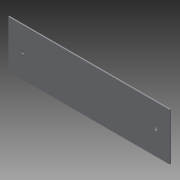
# Autodesk Inventor part: tabliczka z autorami i opiekunem na przod 170 x 50
Saved by Autodesk Inventor 2014 (Build 180170000, 170)
## iProperties
Created: 2018-03-25
Part Number: tabliczka z autorami i opiekunem na przod 170 x 50
Material: Generic
Document SubType Name: Modeling
Designer: HP820
Density: 1 g/cm^3
Appearance: Default
Author: HP820
Autodesk Inventor part; units mm, degrees
(part 1 of 3)
ref_plane "YZ Plane" through (0, 0, 0) normal (1, 0, 0) x (0, 1, 0)
ref_plane "XZ Plane" through (0, 0, 0) normal (0, 1, 0) x (-1, 0, 0)
ref_plane "XY Plane" through (0, 0, 0) normal (0, 0, 1) x (1, 0, 0)
sketch "Sketch1" plane through (0, 0, 0) normal (0, 1, 0) x (-1, 0, 0)
  line L0 (-85, 25) -> (85, 25)
  line L1 (85, 25) -> (85, -25)
  line L2 (85, -25) -> (-85, -25)
  line L3 (-85, -25) -> (-85, 25)
  line L4 (-85, 25) -> (85, -25) construction
  line L5 (85, 25) -> (-85, -25) construction
  point P0 (0, 0)
  dimension "d0" = 170
  dimension "d1" = 50
  constraints: 12 end point, 2 midpoint, 2 parallel, 1 horizontal, 1 perpendicular
  measures "d0" distance of L1.end L2.end
  measures "d1" distance of L0.end L1.end
extrude "Extrusion1" add sketch "Sketch1" along normal blind 1.2
sketch "Sketch2" plane through (0, 1.2, 0) normal (0, 1, 0) x (1, 0, 0)
  line L0 (-82.9131, 23.4055) -> (83.5665, 23.4055) construction
  line L1 (83.5665, 23.4055) -> (83.5665, -23.9623) construction
  line L2 (83.5665, -23.9623) -> (-82.9131, -23.9623) construction
  line L3 (-82.9131, -23.9623) -> (-82.9131, 23.4055) construction
  spline S0 degree 2 poles (-28.4034, 19.5042) (-28.4034, 19.1209) (-28.6486, 18.4256) (-28.8759, 18.1938) knots 0 0 0 1 2 2 2
  spline S1 degree 2 poles (-28.8759, 18.1938) (-29.0141, 18.0467) (-29.3528, 17.8061) (-29.5534, 17.7214) knots 0 0 0 1 2 2 2
  spline S2 degree 2 poles (-29.5534, 17.7214) (-29.7584, 17.6367) (-30.2353, 17.5386) (-30.5295, 17.5386) knots 0 0 0 1 2 2 2
  line L4 (-30.5295, 17.5386) -> (-31.2515, 17.5386)
  line L5 (-31.2515, 17.5386) -> (-31.2515, 15.738)
  line L6 (-31.2515, 15.738) -> (-32.6332, 15.738)
  line L7 (-32.6332, 15.738) -> (-32.6332, 21.238)
  line L8 (-32.6332, 21.238) -> (-30.4983, 21.238)
  spline S3 degree 2 poles (-30.4983, 21.238) (-30.0258, 21.238) (-29.335, 21.0642) (-29.0542, 20.877) knots 0 0 0 1 2 2 2
  spline S4 degree 2 poles (-29.0542, 20.877) (-28.7422, 20.6675) (-28.4034, 19.9811) (-28.4034, 19.5042) knots 0 0 0 1 2 2 2
  spline S5 degree 2 poles (-29.8208, 19.4685) (-29.8208, 19.7048) (-30.0436, 20.039) (-30.1952, 20.1014) knots 0 0 0 1 2 2 2
  spline S6 degree 2 poles (-30.1952, 20.1014) (-30.3913, 20.1861) (-30.7479, 20.2129) (-31.0554, 20.2129) knots 0 0 0 1 2 2 2
  line L9 (-31.0554, 20.2129) -> (-31.2515, 20.2129)
  line L10 (-31.2515, 20.2129) -> (-31.2515, 18.5638)
  line L11 (-31.2515, 18.5638) -> (-31.1534, 18.5638)
  spline S7 degree 2 poles (-31.1534, 18.5638) (-30.9618, 18.5638) (-30.6141, 18.5727) (-30.4849, 18.595) knots 0 0 0 1 2 2 2
  spline S8 degree 2 poles (-30.4849, 18.595) (-30.3735, 18.6128) (-30.1283, 18.7197) (-30.0615, 18.7866) knots 0 0 0 1 2 2 2
  spline S9 degree 2 poles (-30.0615, 18.7866) (-29.9188, 18.9203) (-29.8208, 19.2189) (-29.8208, 19.4685) knots 0 0 0 1 2 2 2
  line L12 (-24.9537, 18.6618) -> (-25.0607, 18.6618)
  spline S10 degree 2 poles (-25.0607, 18.6618) (-25.1364, 18.6886) (-25.4172, 18.7153) (-25.5866, 18.7153) knots 0 0 0 1 2 2 2
  spline S11 degree 2 poles (-25.5866, 18.7153) (-25.7872, 18.7153) (-26.2373, 18.595) (-26.4468, 18.5147) knots 0 0 0 1 2 2 2
  line L13 (-26.4468, 18.5147) -> (-26.4468, 15.738)
  line L14 (-26.4468, 15.738) -> (-27.7393, 15.738)
  line L15 (-27.7393, 15.738) -> (-27.7393, 19.8875)
  line L16 (-27.7393, 19.8875) -> (-26.4468, 19.8875)
  line L17 (-26.4468, 19.8875) -> (-26.4468, 19.2903)
  spline S12 degree 2 poles (-26.4468, 19.2903) (-26.3577, 19.3705) (-26.0457, 19.6201) (-25.9164, 19.6958) knots 0 0 0 1 2 2 2
  spline S13 degree 2 poles (-25.9164, 19.6958) (-25.7738, 19.7805) (-25.3994, 19.9009) (-25.2345, 19.9009) knots 0 0 0 1 2 2 2
  spline S14 degree 2 poles (-25.2345, 19.9009) (-25.1721, 19.9009) (-25.0161, 19.892) (-24.9537, 19.8875) knots 0 0 0 1 2 2 2
  line L18 (-24.9537, 19.8875) -> (-24.9537, 18.6618)
  spline S15 degree 2 poles (-20.4788, 17.8105) (-20.4788, 16.7854) (-21.5975, 15.6087) (-22.6182, 15.6087) knots 0 0 0 1 2 2 2
  spline S16 degree 2 poles (-22.6182, 15.6087) (-23.6344, 15.6087) (-24.762, 16.7854) (-24.762, 17.8105) knots 0 0 0 1 2 2 2
  spline S17 degree 2 poles (-24.762, 17.8105) (-24.762, 18.8445) (-23.6344, 20.0168) (-22.6182, 20.0168) knots 0 0 0 1 2 2 2
  spline S18 degree 2 poles (-22.6182, 20.0168) (-21.602, 20.0168) (-20.4788, 18.8401) (-20.4788, 17.8105) knots 0 0 0 1 2 2 2
  spline S19 degree 2 poles (-21.8026, 17.8016) (-21.8026, 18.1715) (-21.9229, 18.6663) (-22.0299, 18.8133) knots 0 0 0 1 2 2 2
  spline S20 degree 2 poles (-22.0299, 18.8133) (-22.1457, 18.9693) (-22.4355, 19.0897) (-22.6182, 19.0897) knots 0 0 0 1 2 2 2
  spline S21 degree 2 poles (-22.6182, 19.0897) (-22.7965, 19.0897) (-23.0773, 18.9827) (-23.1932, 18.8312) knots 0 0 0 1 2 2 2
  spline S22 degree 2 poles (-23.1932, 18.8312) (-23.3046, 18.6886) (-23.4383, 18.1849) (-23.4383, 17.8016) knots 0 0 0 1 2 2 2
  spline S23 degree 2 poles (-23.4383, 17.8016) (-23.4383, 17.4227) (-23.3135, 16.9548) (-23.211, 16.8121) knots 0 0 0 1 2 2 2
  spline S24 degree 2 poles (-23.211, 16.8121) (-23.1085, 16.6695) (-22.7965, 16.5358) (-22.6093, 16.5358) knots 0 0 0 1 2 2 2
  spline S25 degree 2 poles (-22.6093, 16.5358) (-22.4533, 16.5358) (-22.1324, 16.6695) (-22.0343, 16.8032) knots 0 0 0 1 2 2 2
  spline S26 degree 2 poles (-22.0343, 16.8032) (-21.9229, 16.9592) (-21.8026, 17.4094) (-21.8026, 17.8016) knots 0 0 0 1 2 2 2
  spline S27 degree 2 poles (-18.0363, 15.6667) (-18.0363, 14.9625) (-18.8698, 14.178) (-19.5295, 14.178) knots 0 0 0 1 2 2 2
  spline S28 degree 2 poles (-19.5295, 14.178) (-19.886, 14.178) (-20.461, 14.2404) (-20.5947, 14.2761) knots 0 0 0 1 2 2 2
  line L19 (-20.5947, 14.2761) -> (-20.5947, 15.2299)
  line L20 (-20.5947, 15.2299) -> (-20.4966, 15.2299)
  spline S29 degree 2 poles (-20.4966, 15.2299) (-20.3674, 15.1898) (-20.0643, 15.1407) (-19.9707, 15.1407) knots 0 0 0 1 2 2 2
  spline S30 degree 2 poles (-19.9707, 15.1407) (-19.5963, 15.1407) (-19.3289, 15.5998) (-19.3289, 16.1213) knots 0 0 0 1 2 2 2
  line L21 (-19.3289, 16.1213) -> (-19.3289, 18.9872)
  line L22 (-19.3289, 18.9872) -> (-20.0732, 18.9872)
  line L23 (-20.0732, 18.9872) -> (-20.0732, 19.8875)
  line L24 (-20.0732, 19.8875) -> (-18.0363, 19.8875)
  line L25 (-18.0363, 19.8875) -> (-18.0363, 15.6667)
  line L26 (-18.0363, 20.4803) -> (-19.4136, 20.4803)
  line L27 (-19.4136, 20.4803) -> (-19.4136, 21.4876)
  line L28 (-19.4136, 21.4876) -> (-18.0363, 21.4876)
  line L29 (-18.0363, 21.4876) -> (-18.0363, 20.4803)
  spline S31 degree 2 poles (-14.9209, 15.6266) (-16.0975, 15.6266) (-17.35, 16.7497) (-17.35, 17.7882) knots 0 0 0 1 2 2 2
  spline S32 degree 2 poles (-17.35, 17.7882) (-17.35, 18.8044) (-16.1822, 20.0168) (-15.1303, 20.0168) knots 0 0 0 1 2 2 2
  spline S33 degree 2 poles (-15.1303, 20.0168) (-14.181, 20.0168) (-13.2183, 18.9872) (-13.2183, 18.0334) knots 0 0 0 1 2 2 2
  line L30 (-13.2183, 18.0334) -> (-13.2183, 17.5654)
  line L31 (-13.2183, 17.5654) -> (-16.0574, 17.5654)
  spline S34 degree 2 poles (-16.0574, 17.5654) (-16.0396, 17.2757) (-15.8301, 16.8924) (-15.6607, 16.7765) knots 0 0 0 1 2 2 2
  spline S35 degree 2 poles (-15.6607, 16.7765) (-15.4958, 16.6606) (-15.0501, 16.5625) (-14.7872, 16.5625) knots 0 0 0 1 2 2 2
  spline S36 degree 2 poles (-14.7872, 16.5625) (-14.5643, 16.5625) (-14.1275, 16.6606) (-13.9448, 16.7453) knots 0 0 0 1 2 2 2
  spline S37 degree 2 poles (-13.9448, 16.7453) (-13.7843, 16.8121) (-13.5169, 16.977) (-13.4322, 17.0394) knots 0 0 0 1 2 2 2
  line L32 (-13.4322, 17.0394) -> (-13.294, 17.0394)
  line L33 (-13.294, 17.0394) -> (-13.294, 15.9697)
  spline S38 degree 2 poles (-13.294, 15.9697) (-13.4545, 15.9074) (-13.713, 15.8004) (-13.9448, 15.7469) knots 0 0 0 1 2 2 2
  spline S39 degree 2 poles (-13.9448, 15.7469) (-14.1543, 15.689) (-14.6, 15.6266) (-14.9209, 15.6266) knots 0 0 0 1 2 2 2
  spline S40 degree 2 poles (-14.493, 18.3454) (-14.5019, 18.7554) (-14.8629, 19.1877) (-15.2329, 19.1877) knots 0 0 0 1 2 2 2
  spline S41 degree 2 poles (-15.2329, 19.1877) (-15.6117, 19.1877) (-16.0396, 18.7331) (-16.0619, 18.3454) knots 0 0 0 1 2 2 2
  line L34 (-16.0619, 18.3454) -> (-14.493, 18.3454)
  line L35 (-8.4002, 15.738) -> (-9.9379, 15.738)
  line L36 (-9.9379, 15.738) -> (-11.0611, 17.5386)
  line L37 (-11.0611, 17.5386) -> (-11.2616, 17.2712)
  line L38 (-11.2616, 17.2712) -> (-11.2616, 15.738)
  line L39 (-11.2616, 15.738) -> (-12.5542, 15.738)
  line L40 (-12.5542, 15.738) -> (-12.5542, 21.4831)
  line L41 (-12.5542, 21.4831) -> (-11.2616, 21.4831)
  line L42 (-11.2616, 21.4831) -> (-11.2616, 18.2651)
  line L43 (-11.2616, 18.2651) -> (-10.0359, 19.8875)
  line L44 (-10.0359, 19.8875) -> (-8.5072, 19.8875)
  line L45 (-8.5072, 19.8875) -> (-9.9602, 18.1002)
  line L46 (-9.9602, 18.1002) -> (-8.4002, 15.738)
  spline S42 degree 2 poles (-6.4079, 15.6578) (-7.1968, 15.6578) (-7.9188, 16.3085) (-7.9188, 17.0484) knots 0 0 0 1 2 2 2
  line L47 (-7.9188, 17.0484) -> (-7.9188, 18.9872)
  line L48 (-7.9188, 18.9872) -> (-8.4136, 18.9872)
  line L49 (-8.4136, 18.9872) -> (-8.4136, 19.8875)
  line L50 (-8.4136, 19.8875) -> (-7.9188, 19.8875)
  line L51 (-7.9188, 19.8875) -> (-7.9188, 21.0731)
  line L52 (-7.9188, 21.0731) -> (-6.6263, 21.0731)
  line L53 (-6.6263, 21.0731) -> (-6.6263, 19.8875)
  line L54 (-6.6263, 19.8875) -> (-5.3783, 19.8875)
  line L55 (-5.3783, 19.8875) -> (-5.3783, 18.9872)
  line L56 (-5.3783, 18.9872) -> (-6.6263, 18.9872)
  line L57 (-6.6263, 18.9872) -> (-6.6263, 17.5119)
  spline S43 degree 2 poles (-6.6263, 17.5119) (-6.6263, 17.2935) (-6.6174, 16.9681) (-6.5639, 16.8389) knots 0 0 0 1 2 2 2
  spline S44 degree 2 poles (-6.5639, 16.8389) (-6.5104, 16.7096) (-6.2474, 16.5581) (-5.9979, 16.5581) knots 0 0 0 1 2 2 2
  spline S45 degree 2 poles (-5.9979, 16.5581) (-5.8909, 16.5581) (-5.5566, 16.6472) (-5.4897, 16.6829) knots 0 0 0 1 2 2 2
  line L58 (-5.4897, 16.6829) -> (-5.3783, 16.6829)
  line L59 (-5.3783, 16.6829) -> (-5.3783, 15.7736)
  spline S46 degree 2 poles (-5.3783, 15.7736) (-5.5878, 15.7202) (-6.0602, 15.6578) (-6.4079, 15.6578) knots 0 0 0 1 2 2 2
  line L60 (3.5447, 19.8875) -> (2.3324, 15.738)
  line L61 (2.3324, 15.738) -> (0.9596, 15.738)
  line L62 (0.9596, 15.738) -> (0.2286, 18.4211)
  line L63 (0.2286, 18.4211) -> (-0.5023, 15.738)
  line L64 (-0.5023, 15.738) -> (-1.8751, 15.738)
  line L65 (-1.8751, 15.738) -> (-3.0785, 19.8875)
  line L66 (-3.0785, 19.8875) -> (-1.7191, 19.8875)
  line L67 (-1.7191, 19.8875) -> (-1.0817, 17.142)
  line L68 (-1.0817, 17.142) -> (-0.2973, 19.8875)
  line L69 (-0.2973, 19.8875) -> (0.8482, 19.8875)
  line L70 (0.8482, 19.8875) -> (1.588, 17.142)
  line L71 (1.588, 17.142) -> (2.2165, 19.8875)
  line L72 (2.2165, 19.8875) -> (3.5447, 19.8875)
  line L73 (7.9616, 19.8875) -> (5.8713, 14.2181)
  line L74 (5.8713, 14.2181) -> (4.4807, 14.2181)
  line L75 (4.4807, 14.2181) -> (5.1091, 15.8405)
  line L76 (5.1091, 15.8405) -> (3.5893, 19.8875)
  line L77 (3.5893, 19.8875) -> (4.9442, 19.8875)
  line L78 (4.9442, 19.8875) -> (5.8178, 17.2846)
  line L79 (5.8178, 17.2846) -> (6.6334, 19.8875)
  line L80 (6.6334, 19.8875) -> (7.9616, 19.8875)
  line L81 (12.6014, 15.738) -> (11.0637, 15.738)
  line L82 (11.0637, 15.738) -> (9.9406, 17.5386)
  line L83 (9.9406, 17.5386) -> (9.74, 17.2712)
  line L84 (9.74, 17.2712) -> (9.74, 15.738)
  line L85 (9.74, 15.738) -> (8.4474, 15.738)
  line L86 (8.4474, 15.738) -> (8.4474, 21.4831)
  line L87 (8.4474, 21.4831) -> (9.74, 21.4831)
  line L88 (9.74, 21.4831) -> (9.74, 18.2651)
  line L89 (9.74, 18.2651) -> (10.9657, 19.8875)
  line L90 (10.9657, 19.8875) -> (12.4945, 19.8875)
  line L91 (12.4945, 19.8875) -> (11.0415, 18.1002)
  line L92 (11.0415, 18.1002) -> (12.6014, 15.738)
  spline S47 degree 2 poles (16.9872, 17.8105) (16.9872, 16.7854) (15.8684, 15.6087) (14.8478, 15.6087) knots 0 0 0 1 2 2 2
  spline S48 degree 2 poles (14.8478, 15.6087) (13.8316, 15.6087) (12.7039, 16.7854) (12.7039, 17.8105) knots 0 0 0 1 2 2 2
  spline S49 degree 2 poles (12.7039, 17.8105) (12.7039, 18.8445) (13.8316, 20.0168) (14.8478, 20.0168) knots 0 0 0 1 2 2 2
  spline S50 degree 2 poles (14.8478, 20.0168) (15.864, 20.0168) (16.9872, 18.8401) (16.9872, 17.8105) knots 0 0 0 1 2 2 2
  spline S51 degree 2 poles (15.6634, 17.8016) (15.6634, 18.1715) (15.5431, 18.6663) (15.4361, 18.8133) knots 0 0 0 1 2 2 2
  spline S52 degree 2 poles (15.4361, 18.8133) (15.3202, 18.9693) (15.0305, 19.0897) (14.8478, 19.0897) knots 0 0 0 1 2 2 2
  spline S53 degree 2 poles (14.8478, 19.0897) (14.6695, 19.0897) (14.3887, 18.9827) (14.2728, 18.8312) knots 0 0 0 1 2 2 2
  spline S54 degree 2 poles (14.2728, 18.8312) (14.1614, 18.6886) (14.0277, 18.1849) (14.0277, 17.8016) knots 0 0 0 1 2 2 2
  spline S55 degree 2 poles (14.0277, 17.8016) (14.0277, 17.4227) (14.1525, 16.9548) (14.255, 16.8121) knots 0 0 0 1 2 2 2
  spline S56 degree 2 poles (14.255, 16.8121) (14.3575, 16.6695) (14.6695, 16.5358) (14.8567, 16.5358) knots 0 0 0 1 2 2 2
  spline S57 degree 2 poles (14.8567, 16.5358) (15.0127, 16.5358) (15.3336, 16.6695) (15.4316, 16.8032) knots 0 0 0 1 2 2 2
  spline S58 degree 2 poles (15.4316, 16.8032) (15.5431, 16.9592) (15.6634, 17.4094) (15.6634, 17.8016) knots 0 0 0 1 2 2 2
  line L93 (21.5556, 15.738) -> (20.2542, 15.738)
  line L94 (20.2542, 15.738) -> (20.2542, 17.7927)
  spline S59 degree 2 poles (20.2542, 17.7927) (20.2542, 18.0467) (20.2141, 18.5459) (20.1606, 18.6618) knots 0 0 0 1 2 2 2
  spline S60 degree 2 poles (20.1606, 18.6618) (20.0937, 18.8044) (19.8441, 18.9248) (19.6302, 18.9248) knots 0 0 0 1 2 2 2
  spline S61 degree 2 poles (19.6302, 18.9248) (19.4742, 18.9248) (19.1488, 18.8044) (18.9661, 18.6752) knots 0 0 0 1 2 2 2
  line L95 (18.9661, 18.6752) -> (18.9661, 15.738)
  line L96 (18.9661, 15.738) -> (17.6735, 15.738)
  line L97 (17.6735, 15.738) -> (17.6735, 19.8875)
  line L98 (17.6735, 19.8875) -> (18.9661, 19.8875)
  line L99 (18.9661, 19.8875) -> (18.9661, 19.4284)
  spline S62 degree 2 poles (18.9661, 19.4284) (19.2825, 19.6958) (19.8842, 19.9989) (20.2497, 19.9989) knots 0 0 0 1 2 2 2
  spline S63 degree 2 poles (20.2497, 19.9989) (20.8826, 19.9989) (21.5556, 19.1967) (21.5556, 18.439) knots 0 0 0 1 2 2 2
  line L100 (21.5556, 18.439) -> (21.5556, 15.738)
  spline S64 degree 2 poles (24.8004, 16.1792) (24.6667, 16.0678) (24.4572, 15.8895) (24.2789, 15.8004) knots 0 0 0 1 2 2 2
  spline S65 degree 2 poles (24.2789, 15.8004) (24.1051, 15.7157) (23.7752, 15.6266) (23.4811, 15.6266) knots 0 0 0 1 2 2 2
  spline S66 degree 2 poles (23.4811, 15.6266) (22.9284, 15.6266) (22.2019, 16.3664) (22.2019, 16.928) knots 0 0 0 1 2 2 2
  spline S67 degree 2 poles (22.2019, 16.928) (22.2019, 17.3871) (22.5718, 17.9576) (22.9195, 18.1225) knots 0 0 0 1 2 2 2
  spline S68 degree 2 poles (22.9195, 18.1225) (23.2716, 18.2919) (24.2477, 18.4256) (24.8093, 18.4612) knots 0 0 0 1 2 2 2
  line L101 (24.8093, 18.4612) -> (24.8093, 18.4835)
  spline S69 degree 2 poles (24.8093, 18.4835) (24.8093, 18.8267) (24.3012, 19.0897) (23.7931, 19.0897) knots 0 0 0 1 2 2 2
  spline S70 degree 2 poles (23.7931, 19.0897) (23.5658, 19.0897) (22.9507, 18.9248) (22.661, 18.7955) knots 0 0 0 1 2 2 2
  line L102 (22.661, 18.7955) -> (22.5496, 18.7955)
  line L103 (22.5496, 18.7955) -> (22.5496, 19.7984)
  spline S71 degree 2 poles (22.5496, 19.7984) (22.7412, 19.8518) (23.597, 20.0034) (24.0338, 20.0034) knots 0 0 0 1 2 2 2
  spline S72 degree 2 poles (24.0338, 20.0034) (25.1034, 20.0034) (26.084, 19.2903) (26.084, 18.5593) knots 0 0 0 1 2 2 2
  line L104 (26.084, 18.5593) -> (26.084, 15.738)
  line L105 (26.084, 15.738) -> (24.8004, 15.738)
  line L106 (24.8004, 15.738) -> (24.8004, 16.1792)
  line L107 (24.8004, 16.821) -> (24.8004, 17.6813)
  spline S73 degree 2 poles (24.8004, 17.6813) (24.4705, 17.6501) (24.065, 17.601) (23.8688, 17.5297) knots 0 0 0 1 2 2 2
  spline S74 degree 2 poles (23.8688, 17.5297) (23.695, 17.4718) (23.5078, 17.2311) (23.5078, 17.035) knots 0 0 0 1 2 2 2
  spline S75 degree 2 poles (23.5078, 17.035) (23.5078, 16.7453) (23.8243, 16.5269) (24.1318, 16.5269) knots 0 0 0 1 2 2 2
  spline S76 degree 2 poles (24.1318, 16.5269) (24.3012, 16.5269) (24.6577, 16.6829) (24.8004, 16.821) knots 0 0 0 1 2 2 2
  line L108 (28.3348, 15.738) -> (27.0423, 15.738)
  line L109 (27.0423, 15.738) -> (27.0423, 21.4831)
  line L110 (27.0423, 21.4831) -> (28.3348, 21.4831)
  line L111 (28.3348, 21.4831) -> (28.3348, 15.738)
  line L112 (30.6168, 15.738) -> (29.3243, 15.738)
  line L113 (29.3243, 15.738) -> (29.3243, 19.8875)
  line L114 (29.3243, 19.8875) -> (30.6168, 19.8875)
  line L115 (30.6168, 19.8875) -> (30.6168, 15.738)
  line L116 (30.6569, 20.4803) -> (29.2886, 20.4803)
  line L117 (29.2886, 20.4803) -> (29.2886, 21.4876)
  line L118 (29.2886, 21.4876) -> (30.6569, 21.4876)
  line L119 (30.6569, 21.4876) -> (30.6569, 20.4803)
  line L120 (33.1395, 18.4345) -> (31.8336, 18.4345)
  line L121 (31.8336, 18.4345) -> (31.8336, 19.8875)
  line L122 (31.8336, 19.8875) -> (33.1395, 19.8875)
  line L123 (33.1395, 19.8875) -> (33.1395, 18.4345)
  line L124 (33.1395, 15.738) -> (31.8336, 15.738)
  line L125 (31.8336, 15.738) -> (31.8336, 17.191)
  line L126 (31.8336, 17.191) -> (33.1395, 17.191)
  line L127 (33.1395, 17.191) -> (33.1395, 15.738)
  line L128 (-36.2144, 6.6824) -> (-39.8826, 6.6824)
  line L129 (-39.8826, 6.6824) -> (-39.8826, 8.4295)
  line L130 (-39.8826, 8.4295) -> (-40.511, 8.0551)
  line L131 (-40.511, 8.0551) -> (-40.511, 8.9421)
  line L132 (-40.511, 8.9421) -> (-39.8826, 9.3076)
  line L133 (-39.8826, 9.3076) -> (-39.8826, 12.1824)
  line L134 (-39.8826, 12.1824) -> (-38.5098, 12.1824)
  line L135 (-38.5098, 12.1824) -> (-38.5098, 10.0653)
  line L136 (-38.5098, 10.0653) -> (-37.3242, 10.7739)
  line L137 (-37.3242, 10.7739) -> (-37.3242, 9.887)
  line L138 (-37.3242, 9.887) -> (-38.5098, 9.1872)
  line L139 (-38.5098, 9.1872) -> (-38.5098, 7.7298)
  line L140 (-38.5098, 7.7298) -> (-36.2144, 7.7298)
  line L141 (-36.2144, 7.7298) -> (-36.2144, 6.6824)
  line L142 (-31.7797, 6.6824) -> (-33.0722, 6.6824)
  line L143 (-33.0722, 6.6824) -> (-33.0722, 7.1415)
  spline S77 degree 2 poles (-33.0722, 7.1415) (-33.4065, 6.8607) (-33.9681, 6.5665) (-34.3558, 6.5665) knots 0 0 0 1 2 2 2
  spline S78 degree 2 poles (-34.3558, 6.5665) (-34.9709, 6.5665) (-35.6618, 7.3465) (-35.6618, 8.1309) knots 0 0 0 1 2 2 2
  line L144 (-35.6618, 8.1309) -> (-35.6618, 10.8319)
  line L145 (-35.6618, 10.8319) -> (-34.3603, 10.8319)
  line L146 (-34.3603, 10.8319) -> (-34.3603, 8.7727)
  spline S79 degree 2 poles (-34.3603, 8.7727) (-34.3603, 8.4518) (-34.3291, 8.0418) (-34.2667, 7.9036) knots 0 0 0 1 2 2 2
  spline S80 degree 2 poles (-34.2667, 7.9036) (-34.2043, 7.7744) (-33.9592, 7.6406) (-33.7363, 7.6406) knots 0 0 0 1 2 2 2
  spline S81 degree 2 poles (-33.7363, 7.6406) (-33.6026, 7.6406) (-33.2282, 7.7744) (-33.0722, 7.8902) knots 0 0 0 1 2 2 2
  line L147 (-33.0722, 7.8902) -> (-33.0722, 10.8319)
  line L148 (-33.0722, 10.8319) -> (-31.7797, 10.8319)
  line L149 (-31.7797, 10.8319) -> (-31.7797, 6.6824)
  line L150 (-26.6362, 6.6824) -> (-28.1739, 6.6824)
  line L151 (-28.1739, 6.6824) -> (-29.2971, 8.483)
  line L152 (-29.2971, 8.483) -> (-29.4977, 8.2156)
  line L153 (-29.4977, 8.2156) -> (-29.4977, 6.6824)
  line L154 (-29.4977, 6.6824) -> (-30.7902, 6.6824)
  line L155 (-30.7902, 6.6824) -> (-30.7902, 12.4275)
  line L156 (-30.7902, 12.4275) -> (-29.4977, 12.4275)
  line L157 (-29.4977, 12.4275) -> (-29.4977, 9.2095)
  line L158 (-29.4977, 9.2095) -> (-28.272, 10.8319)
  line L159 (-28.272, 10.8319) -> (-26.7432, 10.8319)
  line L160 (-26.7432, 10.8319) -> (-28.1962, 9.0446)
  line L161 (-28.1962, 9.0446) -> (-26.6362, 6.6824)
  spline S82 degree 2 poles (-23.9442, 7.1236) (-24.0779, 7.0122) (-24.2874, 6.8339) (-24.4656, 6.7448) knots 0 0 0 1 2 2 2
  spline S83 degree 2 poles (-24.4656, 6.7448) (-24.6395, 6.6601) (-24.9693, 6.571) (-25.2635, 6.571) knots 0 0 0 1 2 2 2
  spline S84 degree 2 poles (-25.2635, 6.571) (-25.8161, 6.571) (-26.5426, 7.3108) (-26.5426, 7.8724) knots 0 0 0 1 2 2 2
  spline S85 degree 2 poles (-26.5426, 7.8724) (-26.5426, 8.3315) (-26.1727, 8.902) (-25.825, 9.0669) knots 0 0 0 1 2 2 2
  spline S86 degree 2 poles (-25.825, 9.0669) (-25.4729, 9.2363) (-24.4968, 9.37) (-23.9353, 9.4056) knots 0 0 0 1 2 2 2
  line L162 (-23.9353, 9.4056) -> (-23.9353, 9.4279)
  spline S87 degree 2 poles (-23.9353, 9.4279) (-23.9353, 9.7711) (-24.4434, 10.0341) (-24.9515, 10.0341) knots 0 0 0 1 2 2 2
  spline S88 degree 2 poles (-24.9515, 10.0341) (-25.1788, 10.0341) (-25.7938, 9.8692) (-26.0835, 9.7399) knots 0 0 0 1 2 2 2
  line L163 (-26.0835, 9.7399) -> (-26.195, 9.7399)
  line L164 (-26.195, 9.7399) -> (-26.195, 10.7428)
  spline S89 degree 2 poles (-26.195, 10.7428) (-26.0033, 10.7962) (-25.1476, 10.9478) (-24.7108, 10.9478) knots 0 0 0 1 2 2 2
  spline S90 degree 2 poles (-24.7108, 10.9478) (-23.6411, 10.9478) (-22.6605, 10.2346) (-22.6605, 9.5037) knots 0 0 0 1 2 2 2
  line L165 (-22.6605, 9.5037) -> (-22.6605, 6.6824)
  line L166 (-22.6605, 6.6824) -> (-23.9442, 6.6824)
  line L167 (-23.9442, 6.6824) -> (-23.9442, 7.1236)
  line L168 (-23.9442, 7.7654) -> (-23.9442, 8.6257)
  spline S91 degree 2 poles (-23.9442, 8.6257) (-24.274, 8.5945) (-24.6796, 8.5454) (-24.8757, 8.4741) knots 0 0 0 1 2 2 2
  spline S92 degree 2 poles (-24.8757, 8.4741) (-25.0495, 8.4162) (-25.2367, 8.1755) (-25.2367, 7.9794) knots 0 0 0 1 2 2 2
  spline S93 degree 2 poles (-25.2367, 7.9794) (-25.2367, 7.6897) (-24.9203, 7.4713) (-24.6127, 7.4713) knots 0 0 0 1 2 2 2
  spline S94 degree 2 poles (-24.6127, 7.4713) (-24.4434, 7.4713) (-24.0868, 7.6273) (-23.9442, 7.7654) knots 0 0 0 1 2 2 2
  spline S95 degree 2 poles (-20.4409, 6.571) (-20.8955, 6.571) (-21.7112, 6.7715) (-21.9786, 6.9052) knots 0 0 0 1 2 2 2
  line L169 (-21.9786, 6.9052) -> (-21.9786, 7.9972)
  line L170 (-21.9786, 7.9972) -> (-21.8716, 7.9972)
  spline S96 degree 2 poles (-21.8716, 7.9972) (-21.778, 7.9259) (-21.5418, 7.7565) (-21.3323, 7.6629) knots 0 0 0 1 2 2 2
  spline S97 degree 2 poles (-21.3323, 7.6629) (-21.1496, 7.5782) (-20.6994, 7.4579) (-20.432, 7.4579) knots 0 0 0 1 2 2 2
  spline S98 degree 2 poles (-20.432, 7.4579) (-20.1601, 7.4579) (-19.7412, 7.6273) (-19.7412, 7.81) knots 0 0 0 1 2 2 2
  spline S99 degree 2 poles (-19.7412, 7.81) (-19.7412, 7.9526) (-19.9328, 8.1042) (-20.2092, 8.1666) knots 0 0 0 1 2 2 2
  spline S100 degree 2 poles (-20.2092, 8.1666) (-20.3562, 8.2067) (-20.8064, 8.2914) (-20.9802, 8.3449) knots 0 0 0 1 2 2 2
  spline S101 degree 2 poles (-20.9802, 8.3449) (-21.4705, 8.4964) (-21.9608, 9.0892) (-21.9608, 9.575) knots 0 0 0 1 2 2 2
  spline S102 degree 2 poles (-21.9608, 9.575) (-21.9608, 9.8513) (-21.7067, 10.3416) (-21.4571, 10.5333) knots 0 0 0 1 2 2 2
  spline S103 degree 2 poles (-21.4571, 10.5333) (-21.212, 10.7205) (-20.4855, 10.9433) (-20.0264, 10.9433) knots 0 0 0 1 2 2 2
  spline S104 degree 2 poles (-20.0264, 10.9433) (-19.5896, 10.9433) (-18.8587, 10.7695) (-18.6091, 10.6492) knots 0 0 0 1 2 2 2
  line L171 (-18.6091, 10.6492) -> (-18.6091, 9.5973)
  line L172 (-18.6091, 9.5973) -> (-18.7116, 9.5973)
  spline S105 degree 2 poles (-18.7116, 9.5973) (-18.7784, 9.6508) (-19.0682, 9.8246) (-19.2019, 9.887) knots 0 0 0 1 2 2 2
  spline S106 degree 2 poles (-19.2019, 9.887) (-19.3668, 9.9583) (-19.7679, 10.0564) (-19.9774, 10.0564) knots 0 0 0 1 2 2 2
  spline S107 degree 2 poles (-19.9774, 10.0564) (-20.2582, 10.0564) (-20.6459, 9.8647) (-20.6459, 9.7087) knots 0 0 0 1 2 2 2
  spline S108 degree 2 poles (-20.6459, 9.7087) (-20.6459, 9.5661) (-20.4543, 9.4056) (-20.1334, 9.3254) knots 0 0 0 1 2 2 2
  spline S109 degree 2 poles (-20.1334, 9.3254) (-19.9685, 9.2853) (-19.5361, 9.2095) (-19.3356, 9.1427) knots 0 0 0 1 2 2 2
  spline S110 degree 2 poles (-19.3356, 9.1427) (-18.8899, 9) (-18.4263, 8.4429) (-18.4263, 7.9794) knots 0 0 0 1 2 2 2
  spline S111 degree 2 poles (-18.4263, 7.9794) (-18.4263, 7.6897) (-18.6982, 7.1593) (-18.9523, 6.981) knots 0 0 0 1 2 2 2
  spline S112 degree 2 poles (-18.9523, 6.981) (-19.2152, 6.7849) (-19.9373, 6.571) (-20.4409, 6.571) knots 0 0 0 1 2 2 2
  line L173 (-14.5041, 6.6824) -> (-18.1277, 6.6824)
  line L174 (-18.1277, 6.6824) -> (-18.1277, 7.5337)
  line L175 (-18.1277, 7.5337) -> (-16.1488, 9.8603)
  line L176 (-16.1488, 9.8603) -> (-18.0386, 9.8603)
  line L177 (-18.0386, 9.8603) -> (-18.0386, 10.8319)
  line L178 (-18.0386, 10.8319) -> (-14.5442, 10.8319)
  line L179 (-14.5442, 10.8319) -> (-14.5442, 9.994)
  line L180 (-14.5442, 9.994) -> (-16.5276, 7.6718)
  line L181 (-16.5276, 7.6718) -> (-14.5041, 7.6718)
  line L182 (-14.5041, 7.6718) -> (-14.5041, 6.6824)
  line L183 (-6.8335, 6.6824) -> (-8.1618, 6.6824)
  line L184 (-8.1618, 6.6824) -> (-10.2833, 10.5154)
  line L185 (-10.2833, 10.5154) -> (-10.2833, 6.6824)
  line L186 (-10.2833, 6.6824) -> (-11.5447, 6.6824)
  line L187 (-11.5447, 6.6824) -> (-11.5447, 12.1824)
  line L188 (-11.5447, 12.1824) -> (-9.851, 12.1824)
  line L189 (-9.851, 12.1824) -> (-8.0949, 9.0312)
  line L190 (-8.0949, 9.0312) -> (-8.0949, 12.1824)
  line L191 (-8.0949, 12.1824) -> (-6.8335, 12.1824)
  line L192 (-6.8335, 12.1824) -> (-6.8335, 6.6824)
  spline S113 degree 2 poles (-1.8105, 8.7549) (-1.8105, 7.7298) (-2.9292, 6.5531) (-3.9498, 6.5531) knots 0 0 0 1 2 2 2
  spline S114 degree 2 poles (-3.9498, 6.5531) (-4.966, 6.5531) (-6.0937, 7.7298) (-6.0937, 8.7549) knots 0 0 0 1 2 2 2
  spline S115 degree 2 poles (-6.0937, 8.7549) (-6.0937, 9.7889) (-4.966, 10.9611) (-3.9498, 10.9611) knots 0 0 0 1 2 2 2
  spline S116 degree 2 poles (-3.9498, 10.9611) (-2.9336, 10.9611) (-1.8105, 9.7845) (-1.8105, 8.7549) knots 0 0 0 1 2 2 2
  spline S117 degree 2 poles (-3.1342, 8.746) (-3.1342, 9.1159) (-3.2545, 9.6107) (-3.3615, 9.7577) knots 0 0 0 1 2 2 2
  spline S118 degree 2 poles (-3.3615, 9.7577) (-3.4774, 9.9137) (-3.7671, 10.0341) (-3.9498, 10.0341) knots 0 0 0 1 2 2 2
  spline S119 degree 2 poles (-3.9498, 10.0341) (-4.1281, 10.0341) (-4.4089, 9.9271) (-4.5248, 9.7756) knots 0 0 0 1 2 2 2
  spline S120 degree 2 poles (-4.5248, 9.7756) (-4.6362, 9.6329) (-4.7699, 9.1293) (-4.7699, 8.746) knots 0 0 0 1 2 2 2
  spline S121 degree 2 poles (-4.7699, 8.746) (-4.7699, 8.3671) (-4.6451, 7.8992) (-4.5426, 7.7565) knots 0 0 0 1 2 2 2
  spline S122 degree 2 poles (-4.5426, 7.7565) (-4.4401, 7.6139) (-4.1281, 7.4802) (-3.9409, 7.4802) knots 0 0 0 1 2 2 2
  spline S123 degree 2 poles (-3.9409, 7.4802) (-3.7849, 7.4802) (-3.464, 7.6139) (-3.366, 7.7476) knots 0 0 0 1 2 2 2
  spline S124 degree 2 poles (-3.366, 7.7476) (-3.2545, 7.9036) (-3.1342, 8.3538) (-3.1342, 8.746) knots 0 0 0 1 2 2 2
  line L193 (5.0579, 10.8319) -> (3.8455, 6.6824)
  line L194 (3.8455, 6.6824) -> (2.4728, 6.6824)
  line L195 (2.4728, 6.6824) -> (1.7418, 9.3655)
  line L196 (1.7418, 9.3655) -> (1.0109, 6.6824)
  line L197 (1.0109, 6.6824) -> (-0.3619, 6.6824)
  line L198 (-0.3619, 6.6824) -> (-1.5653, 10.8319)
  line L199 (-1.5653, 10.8319) -> (-0.2059, 10.8319)
  line L200 (-0.2059, 10.8319) -> (0.4314, 8.0863)
  line L201 (0.4314, 8.0863) -> (1.2159, 10.8319)
  line L202 (1.2159, 10.8319) -> (2.3613, 10.8319)
  line L203 (2.3613, 10.8319) -> (3.1012, 8.0863)
  line L204 (3.1012, 8.0863) -> (3.7297, 10.8319)
  line L205 (3.7297, 10.8319) -> (5.0579, 10.8319)
  spline S125 degree 2 poles (7.8925, 7.1236) (7.7588, 7.0122) (7.5494, 6.8339) (7.3711, 6.7448) knots 0 0 0 1 2 2 2
  spline S126 degree 2 poles (7.3711, 6.7448) (7.1972, 6.6601) (6.8674, 6.571) (6.5733, 6.571) knots 0 0 0 1 2 2 2
  spline S127 degree 2 poles (6.5733, 6.571) (6.0206, 6.571) (5.2941, 7.3108) (5.2941, 7.8724) knots 0 0 0 1 2 2 2
  spline S128 degree 2 poles (5.2941, 7.8724) (5.2941, 8.3315) (5.664, 8.902) (6.0117, 9.0669) knots 0 0 0 1 2 2 2
  spline S129 degree 2 poles (6.0117, 9.0669) (6.3638, 9.2363) (7.3399, 9.37) (7.9015, 9.4056) knots 0 0 0 1 2 2 2
  line L206 (7.9015, 9.4056) -> (7.9015, 9.4279)
  spline S130 degree 2 poles (7.9015, 9.4279) (7.9015, 9.7711) (7.3934, 10.0341) (6.8853, 10.0341) knots 0 0 0 1 2 2 2
  spline S131 degree 2 poles (6.8853, 10.0341) (6.6579, 10.0341) (6.0429, 9.8692) (5.7532, 9.7399) knots 0 0 0 1 2 2 2
  line L207 (5.7532, 9.7399) -> (5.6417, 9.7399)
  line L208 (5.6417, 9.7399) -> (5.6417, 10.7428)
  spline S132 degree 2 poles (5.6417, 10.7428) (5.8334, 10.7962) (6.6891, 10.9478) (7.1259, 10.9478) knots 0 0 0 1 2 2 2
  spline S133 degree 2 poles (7.1259, 10.9478) (8.1956, 10.9478) (9.1762, 10.2346) (9.1762, 9.5037) knots 0 0 0 1 2 2 2
  line L209 (9.1762, 9.5037) -> (9.1762, 6.6824)
  line L210 (9.1762, 6.6824) -> (7.8925, 6.6824)
  line L211 (7.8925, 6.6824) -> (7.8925, 7.1236)
  line L212 (7.8925, 7.7654) -> (7.8925, 8.6257)
  spline S134 degree 2 poles (7.8925, 8.6257) (7.5627, 8.5945) (7.1571, 8.5454) (6.961, 8.4741) knots 0 0 0 1 2 2 2
  spline S135 degree 2 poles (6.961, 8.4741) (6.7872, 8.4162) (6.6, 8.1755) (6.6, 7.9794) knots 0 0 0 1 2 2 2
  spline S136 degree 2 poles (6.6, 7.9794) (6.6, 7.6897) (6.9165, 7.4713) (7.224, 7.4713) knots 0 0 0 1 2 2 2
  spline S137 degree 2 poles (7.224, 7.4713) (7.3934, 7.4713) (7.7499, 7.6273) (7.8925, 7.7654) knots 0 0 0 1 2 2 2
  line L213 (12.9201, 9.6062) -> (12.8131, 9.6062)
  spline S138 degree 2 poles (12.8131, 9.6062) (12.7374, 9.6329) (12.4566, 9.6597) (12.2872, 9.6597) knots 0 0 0 1 2 2 2
  spline S139 degree 2 poles (12.2872, 9.6597) (12.0866, 9.6597) (11.6365, 9.5393) (11.427, 9.4591) knots 0 0 0 1 2 2 2
  line L214 (11.427, 9.4591) -> (11.427, 6.6824)
  line L215 (11.427, 6.6824) -> (10.1344, 6.6824)
  line L216 (10.1344, 6.6824) -> (10.1344, 10.8319)
  line L217 (10.1344, 10.8319) -> (11.427, 10.8319)
  line L218 (11.427, 10.8319) -> (11.427, 10.2346)
  spline S140 degree 2 poles (11.427, 10.2346) (11.5161, 10.3149) (11.8281, 10.5645) (11.9574, 10.6402) knots 0 0 0 1 2 2 2
  spline S141 degree 2 poles (11.9574, 10.6402) (12.1, 10.7249) (12.4744, 10.8453) (12.6393, 10.8453) knots 0 0 0 1 2 2 2
  spline S142 degree 2 poles (12.6393, 10.8453) (12.7017, 10.8453) (12.8577, 10.8363) (12.9201, 10.8319) knots 0 0 0 1 2 2 2
  line L219 (12.9201, 10.8319) -> (12.9201, 9.6062)
  line L220 (17.5688, 6.6824) -> (16.0311, 6.6824)
  line L221 (16.0311, 6.6824) -> (14.9079, 8.483)
  line L222 (14.9079, 8.483) -> (14.7074, 8.2156)
  line L223 (14.7074, 8.2156) -> (14.7074, 6.6824)
  line L224 (14.7074, 6.6824) -> (13.4148, 6.6824)
  line L225 (13.4148, 6.6824) -> (13.4148, 12.4275)
  line L226 (13.4148, 12.4275) -> (14.7074, 12.4275)
  line L227 (14.7074, 12.4275) -> (14.7074, 9.2095)
  line L228 (14.7074, 9.2095) -> (15.9331, 10.8319)
  line L229 (15.9331, 10.8319) -> (17.4618, 10.8319)
  line L230 (17.4618, 10.8319) -> (16.0088, 9.0446)
  line L231 (16.0088, 9.0446) -> (17.5688, 6.6824)
  line L232 (19.2669, 6.6824) -> (17.9744, 6.6824)
  line L233 (17.9744, 6.6824) -> (17.9744, 10.8319)
  line L234 (17.9744, 10.8319) -> (19.2669, 10.8319)
  line L235 (19.2669, 10.8319) -> (19.2669, 6.6824)
  line L236 (19.3071, 11.4247) -> (17.9387, 11.4247)
  line L237 (17.9387, 11.4247) -> (17.9387, 12.432)
  line L238 (17.9387, 12.432) -> (19.3071, 12.432)
  line L239 (19.3071, 12.432) -> (19.3071, 11.4247)
  spline S143 degree 2 poles (22.3824, 6.571) (21.2058, 6.571) (19.9533, 7.6941) (19.9533, 8.7326) knots 0 0 0 1 2 2 2
  spline S144 degree 2 poles (19.9533, 8.7326) (19.9533, 9.7488) (21.1211, 10.9611) (22.1729, 10.9611) knots 0 0 0 1 2 2 2
  spline S145 degree 2 poles (22.1729, 10.9611) (23.1223, 10.9611) (24.085, 9.9316) (24.085, 8.9778) knots 0 0 0 1 2 2 2
  line L240 (24.085, 8.9778) -> (24.085, 8.5098)
  line L241 (24.085, 8.5098) -> (21.2459, 8.5098)
  spline S146 degree 2 poles (21.2459, 8.5098) (21.2637, 8.2201) (21.4732, 7.8368) (21.6425, 7.7209) knots 0 0 0 1 2 2 2
  spline S147 degree 2 poles (21.6425, 7.7209) (21.8075, 7.605) (22.2532, 7.5069) (22.5161, 7.5069) knots 0 0 0 1 2 2 2
  spline S148 degree 2 poles (22.5161, 7.5069) (22.739, 7.5069) (23.1758, 7.605) (23.3585, 7.6897) knots 0 0 0 1 2 2 2
  spline S149 degree 2 poles (23.3585, 7.6897) (23.519, 7.7565) (23.7864, 7.9214) (23.8711, 7.9838) knots 0 0 0 1 2 2 2
  line L242 (23.8711, 7.9838) -> (24.0092, 7.9838)
  line L243 (24.0092, 7.9838) -> (24.0092, 6.9141)
  spline S150 degree 2 poles (24.0092, 6.9141) (23.8488, 6.8517) (23.5903, 6.7448) (23.3585, 6.6913) knots 0 0 0 1 2 2 2
  spline S151 degree 2 poles (23.3585, 6.6913) (23.149, 6.6334) (22.7033, 6.571) (22.3824, 6.571) knots 0 0 0 1 2 2 2
  spline S152 degree 2 poles (22.8103, 9.2898) (22.8014, 9.6998) (22.4404, 10.1321) (22.0704, 10.1321) knots 0 0 0 1 2 2 2
  spline S153 degree 2 poles (22.0704, 10.1321) (21.6916, 10.1321) (21.2637, 9.6775) (21.2414, 9.2898) knots 0 0 0 1 2 2 2
  line L244 (21.2414, 9.2898) -> (22.8103, 9.2898)
  line L245 (30.931, 10.8319) -> (29.7187, 6.6824)
  line L246 (29.7187, 6.6824) -> (28.3459, 6.6824)
  line L247 (28.3459, 6.6824) -> (27.615, 9.3655)
  line L248 (27.615, 9.3655) -> (26.884, 6.6824)
  line L249 (26.884, 6.6824) -> (25.5113, 6.6824)
  line L250 (25.5113, 6.6824) -> (24.3079, 10.8319)
  line L251 (24.3079, 10.8319) -> (25.6673, 10.8319)
  line L252 (25.6673, 10.8319) -> (26.3046, 8.0863)
  line L253 (26.3046, 8.0863) -> (27.0891, 10.8319)
  line L254 (27.0891, 10.8319) -> (28.2345, 10.8319)
  line L255 (28.2345, 10.8319) -> (28.9744, 8.0863)
  line L256 (28.9744, 8.0863) -> (29.6028, 10.8319)
  line L257 (29.6028, 10.8319) -> (30.931, 10.8319)
  line L258 (32.7718, 6.6824) -> (31.4793, 6.6824)
  line L259 (31.4793, 6.6824) -> (31.4793, 10.8319)
  line L260 (31.4793, 10.8319) -> (32.7718, 10.8319)
  line L261 (32.7718, 10.8319) -> (32.7718, 6.6824)
  line L262 (32.8119, 11.4247) -> (31.4436, 11.4247)
  line L263 (31.4436, 11.4247) -> (31.4436, 12.432)
  line L264 (31.4436, 12.432) -> (32.8119, 12.432)
  line L265 (32.8119, 12.432) -> (32.8119, 11.4247)
  spline S154 degree 2 poles (35.7937, 6.571) (35.2811, 6.571) (34.4298, 6.8295) (34.1134, 7.0969) knots 0 0 0 1 2 2 2
  spline S155 degree 2 poles (34.1134, 7.0969) (33.8058, 7.3688) (33.4582, 8.1844) (33.4582, 8.7371) knots 0 0 0 1 2 2 2
  spline S156 degree 2 poles (33.4582, 8.7371) (33.4582, 9.3343) (33.8326, 10.1678) (34.1579, 10.4352) knots 0 0 0 1 2 2 2
  spline S157 degree 2 poles (34.1579, 10.4352) (34.4655, 10.6937) (35.3034, 10.9433) (35.758, 10.9433) knots 0 0 0 1 2 2 2
  spline S158 degree 2 poles (35.758, 10.9433) (36.1012, 10.9433) (36.7876, 10.7829) (37.1353, 10.609) knots 0 0 0 1 2 2 2
  line L266 (37.1353, 10.609) -> (37.1353, 9.5037)
  line L267 (37.1353, 9.5037) -> (36.9703, 9.5037)
  spline S159 degree 2 poles (36.9703, 9.5037) (36.8901, 9.5795) (36.6673, 9.7577) (36.5336, 9.8291) knots 0 0 0 1 2 2 2
  spline S160 degree 2 poles (36.5336, 9.8291) (36.3909, 9.9093) (36.0388, 10.0163) (35.8204, 10.0163) knots 0 0 0 1 2 2 2
  spline S161 degree 2 poles (35.8204, 10.0163) (35.3257, 10.0163) (34.7819, 9.3254) (34.7819, 8.7371) knots 0 0 0 1 2 2 2
  spline S162 degree 2 poles (34.7819, 8.7371) (34.7819, 8.1131) (35.3613, 7.498) (35.8427, 7.498) knots 0 0 0 1 2 2 2
  spline S163 degree 2 poles (35.8427, 7.498) (36.0878, 7.498) (36.4533, 7.6094) (36.587, 7.6897) knots 0 0 0 1 2 2 2
  spline S164 degree 2 poles (36.587, 7.6897) (36.7163, 7.7654) (36.9035, 7.9348) (36.9703, 8.0017) knots 0 0 0 1 2 2 2
  line L268 (36.9703, 8.0017) -> (37.1353, 8.0017)
  line L269 (37.1353, 8.0017) -> (37.1353, 6.8919)
  spline S165 degree 2 poles (37.1353, 6.8919) (37.0238, 6.8428) (36.7341, 6.718) (36.5826, 6.6779) knots 0 0 0 1 2 2 2
  spline S166 degree 2 poles (36.5826, 6.6779) (36.3954, 6.6244) (36.0656, 6.571) (35.7937, 6.571) knots 0 0 0 1 2 2 2
  line L270 (41.0575, 6.6824) -> (37.4339, 6.6824)
  line L271 (37.4339, 6.6824) -> (37.4339, 7.5337)
  line L272 (37.4339, 7.5337) -> (39.4128, 9.8603)
  line L273 (39.4128, 9.8603) -> (37.523, 9.8603)
  line L274 (37.523, 9.8603) -> (37.523, 10.8319)
  line L275 (37.523, 10.8319) -> (41.0173, 10.8319)
  line L276 (41.0173, 10.8319) -> (41.0173, 9.994)
  line L277 (41.0173, 9.994) -> (39.034, 7.6718)
  line L278 (39.034, 7.6718) -> (41.0575, 7.6718)
  line L279 (41.0575, 7.6718) -> (41.0575, 6.6824)
  spline S167 degree 2 poles (-27.3092, -0.7598) (-27.3092, -1.1163) (-27.5544, -1.7492) (-27.7995, -1.9721) knots 0 0 0 1 2 2 2
  spline S168 degree 2 poles (-27.7995, -1.9721) (-28.0759, -2.2217) (-28.8291, -2.4579) (-29.3194, -2.4579) knots 0 0 0 1 2 2 2
  spline S169 degree 2 poles (-29.3194, -2.4579) (-29.6848, -2.4579) (-30.3267, -2.4044) (-30.5718, -2.3509) knots 0 0 0 1 2 2 2
  line L280 (-30.5718, -2.3509) -> (-30.5718, -1.2367)
  line L281 (-30.5718, -1.2367) -> (-30.447, -1.2367)
  spline S170 degree 2 poles (-30.447, -1.2367) (-30.2821, -1.3035) (-29.9211, -1.4194) (-29.6358, -1.4194) knots 0 0 0 1 2 2 2
  spline S171 degree 2 poles (-29.6358, -1.4194) (-29.2703, -1.4194) (-28.8737, -1.2144) (-28.7934, -1.0272) knots 0 0 0 1 2 2 2
  spline S172 degree 2 poles (-28.7934, -1.0272) (-28.7088, -0.8445) (-28.6909, -0.372) (-28.6909, -0.0778) knots 0 0 0 1 2 2 2
  line L282 (-28.6909, -0.0778) -> (-28.6909, 2.1284)
  line L283 (-28.6909, 2.1284) -> (-29.9478, 2.1284)
  line L284 (-29.9478, 2.1284) -> (-29.9478, 3.1268)
  line L285 (-29.9478, 3.1268) -> (-27.3092, 3.1268)
  line L286 (-27.3092, 3.1268) -> (-27.3092, -0.7598)
  spline S173 degree 2 poles (-24.0289, -1.932) (-24.1626, -2.0434) (-24.372, -2.2217) (-24.5503, -2.3108) knots 0 0 0 1 2 2 2
  spline S174 degree 2 poles (-24.5503, -2.3108) (-24.7241, -2.3955) (-25.054, -2.4847) (-25.3481, -2.4847) knots 0 0 0 1 2 2 2
  spline S175 degree 2 poles (-25.3481, -2.4847) (-25.9008, -2.4847) (-26.6273, -1.7448) (-26.6273, -1.1832) knots 0 0 0 1 2 2 2
  spline S176 degree 2 poles (-26.6273, -1.1832) (-26.6273, -0.7241) (-26.2574, -0.1536) (-25.9097, 0.0113) knots 0 0 0 1 2 2 2
  spline S177 degree 2 poles (-25.9097, 0.0113) (-25.5576, 0.1807) (-24.5815, 0.3144) (-24.0199, 0.35) knots 0 0 0 1 2 2 2
  line L287 (-24.0199, 0.35) -> (-24.0199, 0.3723)
  spline S178 degree 2 poles (-24.0199, 0.3723) (-24.0199, 0.7155) (-24.528, 0.9785) (-25.0361, 0.9785) knots 0 0 0 1 2 2 2
  spline S179 degree 2 poles (-25.0361, 0.9785) (-25.2635, 0.9785) (-25.8785, 0.8136) (-26.1682, 0.6843) knots 0 0 0 1 2 2 2
  line L288 (-26.1682, 0.6843) -> (-26.2797, 0.6843)
  line L289 (-26.2797, 0.6843) -> (-26.2797, 1.6871)
  spline S180 degree 2 poles (-26.2797, 1.6871) (-26.088, 1.7406) (-25.2323, 1.8922) (-24.7955, 1.8922) knots 0 0 0 1 2 2 2
  spline S181 degree 2 poles (-24.7955, 1.8922) (-23.7258, 1.8922) (-22.7452, 1.179) (-22.7452, 0.4481) knots 0 0 0 1 2 2 2
  line L290 (-22.7452, 0.4481) -> (-22.7452, -2.3732)
  line L291 (-22.7452, -2.3732) -> (-24.0289, -2.3732)
  line L292 (-24.0289, -2.3732) -> (-24.0289, -1.932)
  line L293 (-24.0289, -1.2902) -> (-24.0289, -0.43)
  spline S182 degree 2 poles (-24.0289, -0.43) (-24.3587, -0.4612) (-24.7643, -0.5102) (-24.9604, -0.5815) knots 0 0 0 1 2 2 2
  spline S183 degree 2 poles (-24.9604, -0.5815) (-25.1342, -0.6394) (-25.3214, -0.8801) (-25.3214, -1.0762) knots 0 0 0 1 2 2 2
  spline S184 degree 2 poles (-25.3214, -1.0762) (-25.3214, -1.3659) (-25.0049, -1.5843) (-24.6974, -1.5843) knots 0 0 0 1 2 2 2
  spline S185 degree 2 poles (-24.6974, -1.5843) (-24.528, -1.5843) (-24.1715, -1.4283) (-24.0289, -1.2902) knots 0 0 0 1 2 2 2
  spline S186 degree 2 poles (-19.7545, -2.4847) (-20.2671, -2.4847) (-21.1184, -2.2261) (-21.4348, -1.9587) knots 0 0 0 1 2 2 2
  spline S187 degree 2 poles (-21.4348, -1.9587) (-21.7424, -1.6868) (-22.09, -0.8712) (-22.09, -0.3185) knots 0 0 0 1 2 2 2
  spline S188 degree 2 poles (-22.09, -0.3185) (-22.09, 0.2787) (-21.7156, 1.1122) (-21.3903, 1.3796) knots 0 0 0 1 2 2 2
  spline S189 degree 2 poles (-21.3903, 1.3796) (-21.0827, 1.6381) (-20.2448, 1.8877) (-19.7902, 1.8877) knots 0 0 0 1 2 2 2
  spline S190 degree 2 poles (-19.7902, 1.8877) (-19.447, 1.8877) (-18.7606, 1.7273) (-18.413, 1.5534) knots 0 0 0 1 2 2 2
  line L294 (-18.413, 1.5534) -> (-18.413, 0.4481)
  line L295 (-18.413, 0.4481) -> (-18.5779, 0.4481)
  spline S191 degree 2 poles (-18.5779, 0.4481) (-18.6581, 0.5239) (-18.881, 0.7021) (-19.0147, 0.7735) knots 0 0 0 1 2 2 2
  spline S192 degree 2 poles (-19.0147, 0.7735) (-19.1573, 0.8537) (-19.5094, 0.9606) (-19.7278, 0.9606) knots 0 0 0 1 2 2 2
  spline S193 degree 2 poles (-19.7278, 0.9606) (-20.2225, 0.9606) (-20.7663, 0.2698) (-20.7663, -0.3185) knots 0 0 0 1 2 2 2
  spline S194 degree 2 poles (-20.7663, -0.3185) (-20.7663, -0.9425) (-20.1869, -1.5576) (-19.7055, -1.5576) knots 0 0 0 1 2 2 2
  spline S195 degree 2 poles (-19.7055, -1.5576) (-19.4604, -1.5576) (-19.0949, -1.4462) (-18.9612, -1.3659) knots 0 0 0 1 2 2 2
  spline S196 degree 2 poles (-18.9612, -1.3659) (-18.8319, -1.2902) (-18.6447, -1.1208) (-18.5779, -1.0539) knots 0 0 0 1 2 2 2
  line L296 (-18.5779, -1.0539) -> (-18.413, -1.0539)
  line L297 (-18.413, -1.0539) -> (-18.413, -2.1637)
  spline S197 degree 2 poles (-18.413, -2.1637) (-18.5244, -2.2128) (-18.8141, -2.3376) (-18.9656, -2.3777) knots 0 0 0 1 2 2 2
  spline S198 degree 2 poles (-18.9656, -2.3777) (-19.1528, -2.4312) (-19.4827, -2.4847) (-19.7545, -2.4847) knots 0 0 0 1 2 2 2
  spline S199 degree 2 poles (-15.6719, -2.4847) (-16.8485, -2.4847) (-18.101, -1.3615) (-18.101, -0.323) knots 0 0 0 1 2 2 2
  spline S200 degree 2 poles (-18.101, -0.323) (-18.101, 0.6932) (-16.9332, 1.9055) (-15.8814, 1.9055) knots 0 0 0 1 2 2 2
  spline S201 degree 2 poles (-15.8814, 1.9055) (-14.932, 1.9055) (-13.9693, 0.876) (-13.9693, -0.0778) knots 0 0 0 1 2 2 2
  line L298 (-13.9693, -0.0778) -> (-13.9693, -0.5458)
  line L299 (-13.9693, -0.5458) -> (-16.8084, -0.5458)
  spline S202 degree 2 poles (-16.8084, -0.5458) (-16.7906, -0.8355) (-16.5811, -1.2189) (-16.4118, -1.3347) knots 0 0 0 1 2 2 2
  spline S203 degree 2 poles (-16.4118, -1.3347) (-16.2468, -1.4506) (-15.8011, -1.5487) (-15.5382, -1.5487) knots 0 0 0 1 2 2 2
  spline S204 degree 2 poles (-15.5382, -1.5487) (-15.3153, -1.5487) (-14.8785, -1.4506) (-14.6958, -1.3659) knots 0 0 0 1 2 2 2
  spline S205 degree 2 poles (-14.6958, -1.3659) (-14.5353, -1.2991) (-14.2679, -1.1342) (-14.1832, -1.0718) knots 0 0 0 1 2 2 2
  line L300 (-14.1832, -1.0718) -> (-14.0451, -1.0718)
  line L301 (-14.0451, -1.0718) -> (-14.0451, -2.1415)
  spline S206 degree 2 poles (-14.0451, -2.1415) (-14.2055, -2.2039) (-14.464, -2.3108) (-14.6958, -2.3643) knots 0 0 0 1 2 2 2
  spline S207 degree 2 poles (-14.6958, -2.3643) (-14.9053, -2.4223) (-15.351, -2.4847) (-15.6719, -2.4847) knots 0 0 0 1 2 2 2
  spline S208 degree 2 poles (-15.244, 0.2341) (-15.2529, 0.6442) (-15.6139, 1.0765) (-15.9839, 1.0765) knots 0 0 0 1 2 2 2
  spline S209 degree 2 poles (-15.9839, 1.0765) (-16.3627, 1.0765) (-16.7906, 0.6219) (-16.8129, 0.2341) knots 0 0 0 1 2 2 2
  line L302 (-16.8129, 0.2341) -> (-15.244, 0.2341)
  line L303 (-9.1512, -2.3732) -> (-10.6889, -2.3732)
  line L304 (-10.6889, -2.3732) -> (-11.8121, -0.5726)
  line L305 (-11.8121, -0.5726) -> (-12.0126, -0.84)
  line L306 (-12.0126, -0.84) -> (-12.0126, -2.3732)
  line L307 (-12.0126, -2.3732) -> (-13.3052, -2.3732)
  line L308 (-13.3052, -2.3732) -> (-13.3052, 3.3719)
  line L309 (-13.3052, 3.3719) -> (-12.0126, 3.3719)
  line L310 (-12.0126, 3.3719) -> (-12.0126, 0.1539)
  line L311 (-12.0126, 0.1539) -> (-10.787, 1.7763)
  line L312 (-10.787, 1.7763) -> (-9.2582, 1.7763)
  line L313 (-9.2582, 1.7763) -> (-10.7112, -0.011)
  line L314 (-10.7112, -0.011) -> (-9.1512, -2.3732)
  line L315 (-0.8388, -2.3732) -> (-2.2116, -2.3732)
  line L316 (-2.2116, -2.3732) -> (-2.2116, 1.2726)
  line L317 (-2.2116, 1.2726) -> (-3.21, -1.0807)
  line L318 (-3.21, -1.0807) -> (-4.1549, -1.0807)
  line L319 (-4.1549, -1.0807) -> (-5.1532, 1.2726)
  line L320 (-5.1532, 1.2726) -> (-5.1532, -2.3732)
  line L321 (-5.1532, -2.3732) -> (-6.4547, -2.3732)
  line L322 (-6.4547, -2.3732) -> (-6.4547, 3.1268)
  line L323 (-6.4547, 3.1268) -> (-4.8635, 3.1268)
  line L324 (-4.8635, 3.1268) -> (-3.6423, 0.4124)
  line L325 (-3.6423, 0.4124) -> (-2.43, 3.1268)
  line L326 (-2.43, 3.1268) -> (-0.8388, 3.1268)
  line L327 (-0.8388, 3.1268) -> (-0.8388, -2.3732)
  spline S210 degree 2 poles (2.5129, -1.932) (2.3792, -2.0434) (2.1697, -2.2217) (1.9914, -2.3108) knots 0 0 0 1 2 2 2
  spline S211 degree 2 poles (1.9914, -2.3108) (1.8176, -2.3955) (1.4878, -2.4847) (1.1936, -2.4847) knots 0 0 0 1 2 2 2
  spline S212 degree 2 poles (1.1936, -2.4847) (0.6409, -2.4847) (-0.0856, -1.7448) (-0.0856, -1.1832) knots 0 0 0 1 2 2 2
  spline S213 degree 2 poles (-0.0856, -1.1832) (-0.0856, -0.7241) (0.2844, -0.1536) (0.632, 0.0113) knots 0 0 0 1 2 2 2
  spline S214 degree 2 poles (0.632, 0.0113) (0.9841, 0.1807) (1.9602, 0.3144) (2.5218, 0.35) knots 0 0 0 1 2 2 2
  line L328 (2.5218, 0.35) -> (2.5218, 0.3723)
  spline S215 degree 2 poles (2.5218, 0.3723) (2.5218, 0.7155) (2.0137, 0.9785) (1.5056, 0.9785) knots 0 0 0 1 2 2 2
  spline S216 degree 2 poles (1.5056, 0.9785) (1.2783, 0.9785) (0.6632, 0.8136) (0.3735, 0.6843) knots 0 0 0 1 2 2 2
  line L329 (0.3735, 0.6843) -> (0.2621, 0.6843)
  line L330 (0.2621, 0.6843) -> (0.2621, 1.6871)
  spline S217 degree 2 poles (0.2621, 1.6871) (0.4537, 1.7406) (1.3095, 1.8922) (1.7463, 1.8922) knots 0 0 0 1 2 2 2
  spline S218 degree 2 poles (1.7463, 1.8922) (2.816, 1.8922) (3.7965, 1.179) (3.7965, 0.4481) knots 0 0 0 1 2 2 2
  line L331 (3.7965, 0.4481) -> (3.7965, -2.3732)
  line L332 (3.7965, -2.3732) -> (2.5129, -2.3732)
  line L333 (2.5129, -2.3732) -> (2.5129, -1.932)
  line L334 (2.5129, -1.2902) -> (2.5129, -0.43)
  spline S219 degree 2 poles (2.5129, -0.43) (2.1831, -0.4612) (1.7775, -0.5102) (1.5814, -0.5815) knots 0 0 0 1 2 2 2
  spline S220 degree 2 poles (1.5814, -0.5815) (1.4075, -0.6394) (1.2203, -0.8801) (1.2203, -1.0762) knots 0 0 0 1 2 2 2
  spline S221 degree 2 poles (1.2203, -1.0762) (1.2203, -1.3659) (1.5368, -1.5843) (1.8443, -1.5843) knots 0 0 0 1 2 2 2
  spline S222 degree 2 poles (1.8443, -1.5843) (2.0137, -1.5843) (2.3703, -1.4283) (2.5129, -1.2902) knots 0 0 0 1 2 2 2
  line L335 (7.5404, 0.5506) -> (7.4335, 0.5506)
  spline S223 degree 2 poles (7.4335, 0.5506) (7.3577, 0.5773) (7.0769, 0.6041) (6.9075, 0.6041) knots 0 0 0 1 2 2 2
  spline S224 degree 2 poles (6.9075, 0.6041) (6.707, 0.6041) (6.2568, 0.4837) (6.0473, 0.4035) knots 0 0 0 1 2 2 2
  line L336 (6.0473, 0.4035) -> (6.0473, -2.3732)
  line L337 (6.0473, -2.3732) -> (4.7548, -2.3732)
  line L338 (4.7548, -2.3732) -> (4.7548, 1.7763)
  line L339 (4.7548, 1.7763) -> (6.0473, 1.7763)
  line L340 (6.0473, 1.7763) -> (6.0473, 1.179)
  spline S225 degree 2 poles (6.0473, 1.179) (6.1365, 1.2593) (6.4485, 1.5089) (6.5777, 1.5846) knots 0 0 0 1 2 2 2
  spline S226 degree 2 poles (6.5777, 1.5846) (6.7203, 1.6693) (7.0947, 1.7897) (7.2596, 1.7897) knots 0 0 0 1 2 2 2
  spline S227 degree 2 poles (7.2596, 1.7897) (7.322, 1.7897) (7.478, 1.7807) (7.5404, 1.7763) knots 0 0 0 1 2 2 2
  line L341 (7.5404, 1.7763) -> (7.5404, 0.5506)
  spline S228 degree 2 poles (9.6219, -2.4535) (8.833, -2.4535) (8.1109, -1.8027) (8.1109, -1.0629) knots 0 0 0 1 2 2 2
  line L342 (8.1109, -1.0629) -> (8.1109, 0.876)
  line L343 (8.1109, 0.876) -> (7.6162, 0.876)
  line L344 (7.6162, 0.876) -> (7.6162, 1.7763)
  line L345 (7.6162, 1.7763) -> (8.1109, 1.7763)
  line L346 (8.1109, 1.7763) -> (8.1109, 2.9619)
  line L347 (8.1109, 2.9619) -> (9.4035, 2.9619)
  line L348 (9.4035, 2.9619) -> (9.4035, 1.7763)
  line L349 (9.4035, 1.7763) -> (10.6515, 1.7763)
  line L350 (10.6515, 1.7763) -> (10.6515, 0.876)
  line L351 (10.6515, 0.876) -> (9.4035, 0.876)
  line L352 (9.4035, 0.876) -> (9.4035, -0.5993)
  spline S229 degree 2 poles (9.4035, -0.5993) (9.4035, -0.8177) (9.4124, -1.1431) (9.4659, -1.2723) knots 0 0 0 1 2 2 2
  spline S230 degree 2 poles (9.4659, -1.2723) (9.5194, -1.4016) (9.7823, -1.5531) (10.0319, -1.5531) knots 0 0 0 1 2 2 2
  spline S231 degree 2 poles (10.0319, -1.5531) (10.1389, -1.5531) (10.4732, -1.464) (10.54, -1.4283) knots 0 0 0 1 2 2 2
  line L353 (10.54, -1.4283) -> (10.6515, -1.4283)
  line L354 (10.6515, -1.4283) -> (10.6515, -2.3376)
  spline S232 degree 2 poles (10.6515, -2.3376) (10.442, -2.3911) (9.9695, -2.4535) (9.6219, -2.4535) knots 0 0 0 1 2 2 2
  line L355 (15.0461, 1.7763) -> (12.9558, -3.8931)
  line L356 (12.9558, -3.8931) -> (11.5652, -3.8931)
  line L357 (11.5652, -3.8931) -> (12.1936, -2.2707)
  line L358 (12.1936, -2.2707) -> (10.6737, 1.7763)
  line L359 (10.6737, 1.7763) -> (12.0287, 1.7763)
  line L360 (12.0287, 1.7763) -> (12.9023, -0.8266)
  line L361 (12.9023, -0.8266) -> (13.7179, 1.7763)
  line L362 (13.7179, 1.7763) -> (15.0461, 1.7763)
  line L363 (19.414, -2.3732) -> (18.1126, -2.3732)
  line L364 (18.1126, -2.3732) -> (18.1126, -0.3185)
  spline S233 degree 2 poles (18.1126, -0.3185) (18.1126, -0.0645) (18.0724, 0.4347) (18.019, 0.5506) knots 0 0 0 1 2 2 2
  spline S234 degree 2 poles (18.019, 0.5506) (17.9521, 0.6932) (17.7025, 0.8136) (17.4886, 0.8136) knots 0 0 0 1 2 2 2
  spline S235 degree 2 poles (17.4886, 0.8136) (17.3326, 0.8136) (17.0072, 0.6932) (16.8245, 0.564) knots 0 0 0 1 2 2 2
  line L365 (16.8245, 0.564) -> (16.8245, -2.3732)
  line L366 (16.8245, -2.3732) -> (15.5319, -2.3732)
  line L367 (15.5319, -2.3732) -> (15.5319, 1.7763)
  line L368 (15.5319, 1.7763) -> (16.8245, 1.7763)
  line L369 (16.8245, 1.7763) -> (16.8245, 1.3172)
  spline S236 degree 2 poles (16.8245, 1.3172) (17.1409, 1.5846) (17.7426, 1.8877) (18.1081, 1.8877) knots 0 0 0 1 2 2 2
  spline S237 degree 2 poles (18.1081, 1.8877) (18.741, 1.8877) (19.414, 1.0854) (19.414, 0.3277) knots 0 0 0 1 2 2 2
  line L370 (19.414, 0.3277) -> (19.414, -2.3732)